Autodesk Inventor part; units mm, degrees
(part 2 of 2)
  line L319 (14.915, 90.5568) -> (34.915, 90.5568) construction
  line L320 (16.8181, 104.3086) -> (13.8181, 104.3086)
  line L321 (19.13, 109.0244) -> (13.3499, 109.0244)
  line L322 (13.3499, 109.0244) -> (17.8499, 109.0244) construction
  line L323 (13.3499, 109.0244) -> (11.0999, 105.1272)
  line L324 (13.8181, 104.3086) -> (12.5681, 102.1435)
  line L325 (20.032, 100.4784) -> (16.8181, 104.3086)
  line L326 (24.915, 102.13) -> (19.13, 109.0244)
  line L327 (-85.493, 62.1764) -> (-91.043, 52.5635)
  line L328 (-82.1749, 61.956) -> (-88.459, 51.0717)
  line L329 (-94.743, 40.1874) -> (-88.459, 51.0717)
  line L330 (-96.593, 42.9507) -> (-91.043, 52.5635)
  line L331 (-101.093, 42.9507) -> (-96.593, 42.9507)
  line L332 (-97.243, 40.1874) -> (-94.743, 40.1874)
  line L333 (-100.9047, 29.4878) -> (-103.983, 37.945)
  line L334 (-101.093, 42.9507) -> (-103.343, 39.0535) construction
  line L335 (-103.983, 37.945) -> (-101.093, 42.9507)
  line L336 (-98.743, 37.5894) -> (-97.243, 40.1874)
  line L337 (-97.0329, 32.8909) -> (-98.743, 37.5894)
  line L338 (-80.9047, 29.4878) -> (-100.9047, 29.4878)
  line L339 (-82.0329, 32.8909) -> (-97.0329, 32.8909)
  line L340 (-79.5329, 37.221) -> (-82.0329, 32.8909)
  line L341 (-77.4047, 35.55) -> (-80.9047, 29.4878)
  line L342 (-77.6536, 37.9051) -> (-79.5329, 37.221)
  line L343 (-75.0555, 36.405) -> (-77.4047, 35.55)
  line L344 (-75.0555, 36.405) -> (-76.3055, 34.2399) construction
  line L345 (-75.0555, 36.405) -> (-76.3055, 34.24) construction
  line L346 (-72.0555, 41.6012) -> (-75.0555, 36.405)
  line L347 (-77.6536, 37.9051) -> (-78.6536, 36.173) construction
  line L348 (-74.6536, 43.1012) -> (-77.6536, 37.9051)
  line L349 (-69.0556, 46.7973) -> (-67.8056, 48.9624) construction
  line L350 (-69.0556, 46.7973) -> (-67.8056, 48.9624) construction
  line L351 (-72.0555, 41.6012) -> (-69.0556, 46.7973)
  line L352 (-74.6536, 43.1012) -> (-71.6536, 48.2973)
  line L353 (-69.0556, 46.7973) -> (-69.4897, 49.2593)
  line L354 (-71.6536, 48.2973) -> (-70.6536, 50.0293) construction
  line L355 (-71.6536, 48.2973) -> (-72.0009, 50.2669)
  line L356 (-69.4897, 49.2593) -> (-65.9897, 55.3215)
  line L357 (-72.0009, 50.2669) -> (-69.5009, 54.597)
  line L358 (-69.5009, 54.597) -> (-77.0009, 67.5874)
  line L359 (-65.9897, 55.3215) -> (-75.9897, 72.642)
  line L360 (-70.9671, 58.1952) -> (-60.9671, 75.5157) construction
  line L361 (-81.9249, 66.7192) -> (-83.4249, 64.1211)
  line L362 (-84.853, 71.0792) -> (-87.743, 66.0735)
  line L363 (-87.743, 66.0735) -> (-85.493, 69.9707) construction
  line L364 (-87.743, 66.0735) -> (-85.493, 62.1764)
  line L365 (-83.4249, 64.1211) -> (-82.1749, 61.956)
  line L366 (-77.0009, 67.5874) -> (-81.9249, 66.7192)
  line L367 (-75.9897, 72.642) -> (-84.853, 71.0792)
  line L368 (-96.5929, -42.9509) -> (-91.0429, -52.5638)
  line L369 (-94.743, -40.1876) -> (-88.459, -51.0719)
  line L370 (-82.1749, -61.9562) -> (-88.459, -51.0719)
  line L371 (-85.4929, -62.1767) -> (-91.0429, -52.5638)
  line L372 (-87.7429, -66.0738) -> (-85.4929, -62.1767)
  line L373 (-83.4249, -64.1213) -> (-82.1749, -61.9562)
  line L374 (-75.9896, -72.6422) -> (-84.8529, -71.0794)
  line L375 (-87.7429, -66.0738) -> (-85.4929, -69.9709) construction
  line L376 (-84.8529, -71.0794) -> (-87.7429, -66.0738)
  line L377 (-81.9249, -66.7193) -> (-83.4249, -64.1213)
  line L378 (-77.0009, -67.5876) -> (-81.9249, -66.7193)
  line L379 (-65.9896, -55.3217) -> (-75.9896, -72.6422)
  line L380 (-69.5009, -54.5972) -> (-77.0009, -67.5876)
  line L381 (-72.0009, -50.2671) -> (-69.5009, -54.5972)
  line L382 (-69.4896, -49.2595) -> (-65.9896, -55.3217)
  line L383 (-71.6536, -48.2974) -> (-72.0009, -50.2671)
  line L384 (-69.0555, -46.7975) -> (-69.4896, -49.2595)
  line L385 (-69.0555, -46.7975) -> (-67.8055, -48.9626) construction
  line L386 (-69.0555, -46.7975) -> (-67.8055, -48.9625) construction
  line L387 (-72.0555, -41.6013) -> (-69.0555, -46.7975)
  line L388 (-71.6536, -48.2974) -> (-70.6536, -50.0295) construction
  line L389 (-74.6536, -43.1013) -> (-71.6536, -48.2974)
  line L390 (-75.0555, -36.4052) -> (-76.3055, -34.2402) construction
  line L391 (-75.0555, -36.4052) -> (-76.3055, -34.2402) construction
  line L392 (-72.0555, -41.6013) -> (-75.0555, -36.4052)
  line L393 (-74.6536, -43.1013) -> (-77.6536, -37.9052)
  line L394 (-75.0555, -36.4052) -> (-77.4048, -35.5502)
  line L395 (-77.6536, -37.9052) -> (-78.6536, -36.1732) construction
  line L396 (-77.6536, -37.9052) -> (-79.5329, -37.2212)
  line L397 (-77.4048, -35.5502) -> (-80.9048, -29.488)
  line L398 (-79.5329, -37.2212) -> (-82.0329, -32.8911)
  line L399 (-82.0329, -32.8911) -> (-97.0329, -32.8911)
  line L400 (-80.9048, -29.488) -> (-100.9048, -29.488)
  line L401 (-85.8821, -32.3617) -> (-95.8821, -15.0412) construction
  line L402 (-98.743, -37.5895) -> (-97.243, -40.1876)
  line L403 (-103.9829, -37.9453) -> (-101.0929, -42.9509)
  line L404 (-101.0929, -42.9509) -> (-103.3429, -39.0538) construction
  line L405 (-101.0929, -42.9509) -> (-96.5929, -42.9509)
  line L406 (-97.243, -40.1876) -> (-94.743, -40.1876)
  line L407 (-97.0329, -32.8911) -> (-98.743, -37.5895)
  line L408 (-100.9048, -29.488) -> (-103.9829, -37.9453)
  point P0 (0, -0.0001)
  point P1 (28.4201, -128.6031)
  point P2 (-28.4202, 128.6029)
  point P3 (0, -0.0001)
  point P4 (28.4201, -128.6031)
  point P5 (-28.4202, 128.6029)
  point P6 (129.4403, -39.0089)
  point P7 (-129.4403, 39.0087)
  point P8 (-125.5836, 39.6889)
  point P9 (-28.4202, 128.6029)
  point P10 (28.4201, -128.6031)
  dimension "d890" = 3.2
  dimension "d891" = 3.2
  dimension "d909" = 0
  dimension "d910" = 180
  dimension "d911" = 10
  dimension "d912" = 110
  dimension "d913" = 360
  dimension "d914" = 360
  dimension "d915" = 10.9
  dimension "d916" = 90
  dimension "d917" = 12.76
  dimension "d918" = 120
  dimension "d919" = 8.7
  dimension "d920" = 90
  dimension "d921" = 10.534
  dimension "d922" = 130
  dimension "d923" = 10.5
  dimension "d924" = 3
  dimension "d925" = 6
  dimension "d926" = 2.5
  dimension "d927" = 40
  dimension "d928" = 7
  dimension "d929" = 20
  dimension "d930" = 60
  dimension "d931" = 9
  dimension "d932" = 129.999
  dimension "d933" = 180
  dimension "d934" = 4.5
  dimension "d935" = 120
  dimension "d936" = 3
  dimension "d937" = 2
  dimension "d938" = 40
  dimension "d939" = 5
  dimension "d940" = 140
  dimension "d941" = 15
  dimension "d942" = 120
  dimension "d943" = 5
  dimension "d944" = 110
  dimension "d945" = 3
  dimension "d946" = 130
  dimension "d947" = 2.5
  dimension "d948" = 120
  dimension "d949" = 3
  dimension "d950" = 90
  dimension "d951" = 180
  dimension "d952" = 180
  dimension "d953" = 10
  dimension "d954" = 110
  dimension "d955" = 360
  dimension "d956" = 360
  dimension "d957" = 57.5
  dimension "d958" = 90
  dimension "d959" = 0.6
  dimension "d960" = 0
  dimension "d961" = 3.3
  dimension "d962" = 0.636
  dimension "d963" = 3.3
  dimension "d965" = 360
  constraints: 818 end point, 44 horizontal, 19 equal length, 14 centre point, 4 vertical, 3 parallel, 3 perpendicular, 2 symmetric about line, 743 other
  measures "d890" diameter of A0
  measures "d891" diameter of A1
  measures "d909" distance between parallel lines of L4 L5
  measures "d910" angle of L6 L7
  measures "d911" distance of L6.end L13.end
  measures "d912" angle of L14 L13
  measures "d915" distance of L68.start L68.end
  measures "d916" angle of L68 L69
  measures "d917" distance of L68.end L70.end
  measures "d918" angle of L70 L71
  measures "d919" distance of L70.end L72.end
  measures "d920" angle of L72 L73
  measures "d921" distance of L72.end L74.end
  measures "d922" angle of L74 L75
  measures "d923" distance of L74.end L76.end
  measures "d924" distance of L76.end L77.end
  measures "d925" distance of L78.start L78.end
  measures "d926" distance of L78.end L80.end
  measures "d927" angle of L80 L81
  measures "d928" distance of L80.end L82.end
  measures "d929" distance of L82.end L83.end
  measures "d930" angle of L83 L84
  measures "d931" distance of L83.end L85.end
  measures "d932" angle of L85 L86
  measures "d933" angle of L87 L88
  measures "d934" distance of L87.end L89.end
  measures "d935" angle of L90 L89
  measures "d936" distance of L78.start L106.start
  measures "d937" distance of L106.end L107.end
  measures "d938" angle of L107 L108
  measures "d939" distance of L107.end L109.end
  measures "d940" angle of L109 L107
  measures "d941" distance of L109.end L110.end
  measures "d942" angle of L109 L110
  measures "d943" distance of L110.end L111.end
  measures "d944" angle of L110 L111
  measures "d945" distance of L111.end L112.end
  measures "d946" angle of L111 L112
  measures "d947" distance of L112.end L113.end
  measures "d948" angle of L112 L113
  measures "d949" distance of L4.start L124.end
  measures "d950" angle of L124 L125
  measures "d951" angle of L128 L129
  measures "d952" angle of L131 L132
  measures "d953" distance of L128.end L134.end
  measures "d954" angle of L135 L134
  measures "d957" distance of L67.start L198.end
  measures "d958" angle of L199 L198
  measures "d959" distance of L200.end L201.end
  measures "d960" distance between parallel lines of L201 L202
  measures "d961" diameter of A12
  measures "d962" distance of L198.end L203.end
  measures "d963" diameter of A13
extrude "Extrusion12" add sketch "Sketch3" against normal blind 3 separate body contours L105 L116 L118 L117 L119 L198 L102 L99 L96 L95 | L78 L80 L82 L83 L200 L110 L109 L107 L106 L105 | L83 L85 L87 L200 L112 L111 L110 | L198 L119 L122 L121 L94 L101 L102 | L200 L87 L89 L91 L92 L104 L94 L198 L121 L120 L123 L114 L113 L112 | L128 L134 L164 L163 L162 L160 L159 L169 L158 L157 L155 L154 L168 L153 L152 L150 L149 L167 L148 L147 L145 L144 L166 L143 L142 L140 L139 L165 L138 L136 | L241 L239 L244 L236 L233 L230 L228 L223 L220 L218 L215 L210 L212 L208 L207 L204 | L282 L280 L285 L277 L274 L271 L269 L264 L261 L259 L256 L251 L253 L249 L248 L245 | L323 L321 L326 L318 L315 L312 L310 L305 L302 L300 L297 L292 L294 L290 L289 L286 | L364 L362 L367 L359 L356 L353 L351 L346 L343 L341 L338 L333 L335 L331 L330 L327 | L405 L403 L408 L400 L397 L394 L392 L387 L384 L382 L379 L374 L376 L372 L371 L368
fillet "Fillet12" radius 5 24 edges at (-30.9375, 1.5, 131.6031) (-27.5173, 1.5, 141) (27.5173, 1.5, 141) (30.9375, 1.5, 131.6031) (98.5028, 1.5, 92.5942) (108.3508, 1.5, 94.3307) (135.8681, 1.5, 46.6693) (129.4403, 1.5, 39.0089) (129.4402, 1.5, -39.0088) (135.8681, 1.5, -46.6692) (108.3508, 1.5, -94.3306) (98.5027, 1.5, -92.5941) (30.9374, 1.5, -131.6029) (27.5172, 1.5, -140.9998) (-30.9376, 1.5, -131.6029) (-27.5173, 1.5, -140.9998) (-98.5028, 1.5, -92.5941) (-108.3509, 1.5, -94.3305) (-135.8682, 1.5, -46.6692) (-129.4403, 1.5, -39.0087) (-129.4403, 1.5, 39.0089) (-135.8682, 1.5, 46.6694) (-108.3509, 1.5, 94.3307) (-98.5028, 1.5, 92.5943)
fillet "Fillet13" radius 2 24 edges at (-30.2097, 1.5, -30.6505) (-23.4386, 1.5, -38.72) (-12.9386, 1.5, -38.72) (-11.0102, 1.5, -36.4219) (11.0102, 1.5, -36.4219) (12.9386, 1.5, -38.72) (23.4386, 1.5, -38.72) (30.2097, 1.5, -30.6505) (30.2097, 1.5, -21.9505) (36.5897, 1.5, -10.9001) (36.5897, 1.5, 10.8999) (30.2097, 1.5, 21.9504) (30.2097, 1.5, 30.6504) (23.4386, 1.5, 38.7199) (12.9386, 1.5, 38.7199) (11.0102, 1.5, 36.4218) (-11.0102, 1.5, 36.4218) (-12.9386, 1.5, 38.7199) (-23.4386, 1.5, 38.7199) (-30.2097, 1.5, 30.6504) (-30.2097, 1.5, 21.9504) (-36.5897, 1.5, 10.8999) (-36.5897, 1.5, -10.9001) (-30.2097, 1.5, -21.9505)
body "Solid11"
body "Solid12"
